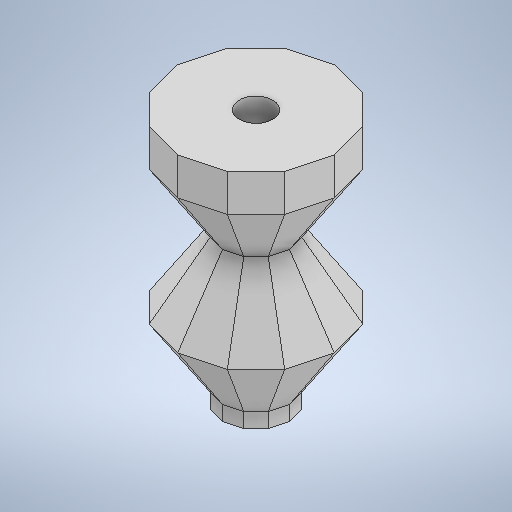
# Autodesk Inventor part: diameter21mm
Saved by Autodesk Inventor 2025.1 (Build 291241000, 241)
## iProperties
Created: 2024-08-09
Part Number: diameter21mm
Material: 일반
Document SubType Name: Modeling
Designer: 82103
Density: 1 g/cm^3
Appearance: 기본값
Author: 82103
Autodesk Inventor part; units mm, degrees
ref_plane "YZ Plane" through (0, 0, 0) normal (1, 0, 0) x (0, 1, 0)
ref_plane "XY Plane" through (0, 0, 0) normal (0, 0, 1) x (1, 0, 0)
sketch "스케치1" plane through (0, 0, 0) normal (0, 1, 0) x (-1, 0, 0)
  line L0 (5.25, -9.0933) -> (0, -10.5)
  line L1 (0, -10.5) -> (-5.25, -9.0933)
  line L2 (-5.25, -9.0933) -> (-9.0933, -5.25)
  line L3 (-9.0933, -5.25) -> (-10.5, 0)
  line L4 (-10.5, 0) -> (-9.0933, 5.25)
  line L5 (-9.0933, 5.25) -> (-5.25, 9.0933)
  line L6 (-5.25, 9.0933) -> (0, 10.5)
  line L7 (0, 10.5) -> (5.25, 9.0933)
  line L8 (5.25, 9.0933) -> (9.0933, 5.25)
  line L9 (9.0933, 5.25) -> (10.5, 0)
  line L10 (10.5, 0) -> (9.0933, -5.25)
  line L11 (9.0933, -5.25) -> (5.25, -9.0933)
  point P0 (0, 0)
  point P1 (0, 0)
  dimension "d0" = 21
  constraints: 24 end point, 1 coincident, 1 horizontal alignment, 25 other
  measures "d0" distance of L3.end L9.end
ref_plane "작업 평면1" through (0, 9, 0) normal (0, 1, 0) x (-1, 0, 0)
sketch "스케치2" plane through (0, 9, 0) normal (0, 1, 0) x (-1, 0, 0)
  line L0 (2.25, -3.8971) -> (0, -4.5)
  line L1 (0, -4.5) -> (-2.25, -3.8971)
  line L2 (-2.25, -3.8971) -> (-3.8971, -2.25)
  line L3 (-3.8971, -2.25) -> (-4.5, 0)
  line L4 (-4.5, 0) -> (-3.8971, 2.25)
  line L5 (-3.8971, 2.25) -> (-2.25, 3.8971)
  line L6 (-2.25, 3.8971) -> (0, 4.5)
  line L7 (0, 4.5) -> (2.25, 3.8971)
  line L8 (2.25, 3.8971) -> (3.8971, 2.25)
  line L9 (3.8971, 2.25) -> (4.5, 0)
  line L10 (4.5, 0) -> (3.8971, -2.25)
  line L11 (3.8971, -2.25) -> (2.25, -3.8971)
  point P0 (0, 0)
  point P1 (0, 0)
  dimension "d2" = 9
  constraints: 24 end point, 1 coincident, 1 horizontal alignment, 25 other
  measures "d2" distance of L3.end L9.end
loft "로프트1" add profiles "스케치2", "스케치1"
mirror "미러1" about plane through (0, 9, 0) normal (0, 1, 0) of "로프트1"
mirror "미러2" about plane through (0, 0, 0) normal (0, 1, 0) of "로프트1"
shell "쉘1" thickness 0.5 removed faces 0 ; own thickness 2 on faces at (-6.4886, -1.5, 6.4886) (-8.8636, -1.5, 2.375) (-8.8636, -1.5, -2.375) (-2.375, -1.5, 8.8636) (-2.375, 16.5, 8.8636) (-6.4886, 16.5, 6.4886) (-8.8636, 16.5, 2.375) (-8.8636, 16.5, -2.375) (-6.4886, -1.5, -6.4886) (-2.375, -1.5, -8.8636) (2.375, -1.5, -8.8636) (6.4886, -1.5, -6.4886) (8.8636, -1.5, -2.375) (8.8636, -1.5, 2.375) (6.4886, -1.5, 6.4886) (2.375, -1.5, 8.8636) (-6.4886, 16.5, -6.4886) (-2.375, 16.5, -8.8636) (2.375, 16.5, -8.8636) (6.4886, 16.5, -6.4886) (8.8636, 16.5, -2.375) (8.8636, 16.5, 2.375) (6.4886, 16.5, 6.4886) (2.375, 16.5, 8.8636)
sketch "스케치3" plane through (-2.25, -9, -3.8971) normal (0, -1, 0) x (0.9659258, 0, -0.258819)
  line L0 (0, 0) -> (2.3294, 0) projected
  line L1 (2.3294, 0) -> (4.3467, 1.1647) projected
  line L2 (4.3467, 1.1647) -> (5.5114, 3.182) projected
  line L3 (5.5114, 3.182) -> (5.5114, 5.5114) projected
  line L4 (5.5114, 5.5114) -> (4.3467, 7.5286) projected
  line L5 (4.3467, 7.5286) -> (2.3294, 8.6933) projected
  line L6 (2.3294, 8.6933) -> (0, 8.6933) projected
  line L7 (0, 8.6933) -> (-2.0173, 7.5286) projected
  line L8 (-2.0173, 7.5286) -> (-3.182, 5.5114) projected
  line L9 (-3.182, 5.5114) -> (-3.182, 3.182) projected
  line L10 (-3.182, 3.182) -> (-2.0173, 1.1647) projected
  line L11 (-2.0173, 1.1647) -> (0, 0) projected
  point P0 (1.1647, 4.3467)
extrude "돌출1" add sketch "스케치3" along normal blind 2
sketch "스케치4" plane through (-5.25, 18, -9.0933) normal (0, 1, 0) x (0.9659258, 0, -0.258819)
  line L0 (0, 0) -> (5.4352, 0) projected
  line L1 (-4.707, -2.7176) -> (0, 0) projected
  line L2 (-7.4246, -7.4246) -> (-4.707, -2.7176) projected
  line L3 (-7.4246, -12.8598) -> (-7.4246, -7.4246) projected
  line L4 (-4.707, -17.5668) -> (-7.4246, -12.8598) projected
  line L5 (0, -20.2844) -> (-4.707, -17.5668) projected
  line L6 (5.4352, -20.2844) -> (0, -20.2844) projected
  line L7 (10.1422, -17.5668) -> (5.4352, -20.2844) projected
  line L8 (12.8598, -12.8598) -> (10.1422, -17.5668) projected
  line L9 (12.8598, -7.4246) -> (12.8598, -12.8598) projected
  line L10 (10.1422, -2.7176) -> (12.8598, -7.4246) projected
  line L11 (5.4352, 0) -> (10.1422, -2.7176) projected
  point P0 (2.7176, -10.1422)
extrude "돌출2" add sketch "스케치4" along normal blind 5
sketch "스케치5" plane through (-5.25, 23, -9.0933) normal (0, 1, 0) x (0.9659258, 0, -0.258819)
  circle A0 centre (2.7176, -10.1422) radius 2.25
  dimension "d13" = 4.5
  constraints: 1 centre point, 1 coincident
  measures "d13" diameter of A0
extrude "돌출3" cut sketch "스케치5" against normal blind 5.5
